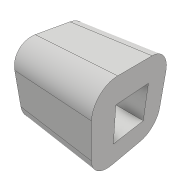
# Autodesk Inventor part: Winding
Saved by Autodesk Inventor 2018.2 (Build 222227000, 227)
## iProperties
Created: 2019-02-04
Part Number: Winding
Material: Generic
Document SubType Name: Modeling
Designer: ns6022
Density: 1 g/cm^3
Appearance: Default
Author: ns6022
Autodesk Inventor part; units mm, degrees
ref_plane "YZ Plane" through (0, 0, 0) normal (1, 0, 0) x (0, 1, 0)
ref_plane "XZ Plane" through (0, 0, 0) normal (0, 1, 0) x (-1, 0, 0)
ref_plane "XY Plane" through (0, 0, 0) normal (0, 0, 1) x (1, 0, 0)
sketch "Sketch1" plane through (0, 0, 0) normal (0, 0, 1) x (1, 0, 0)
  point P0 (0, 0)
sketch "LAYER1" plane through (0, 0, 0) normal (0, 0, 1) x (1, 0, 0)
  line L0 (70, 20.5) -> (90, 20.5)
  line L1 (90, 20.5) -> (90, 57.5)
  line L2 (90, 57.5) -> (0, 57.5)
  line L3 (0, 57.5) -> (0, -57.5)
  line L4 (0, -57.5) -> (90, -57.5)
  line L5 (90, -57.5) -> (90, -20.5)
  line L6 (90, -20.5) -> (70, -20.5)
  line L7 (70, -20.5) -> (70, -37.5)
  line L8 (70, -37.5) -> (20, -37.5)
  line L9 (20, -37.5) -> (20, 37.5)
  line L10 (20, 37.5) -> (70, 37.5)
  line L11 (70, 37.5) -> (70, 20.5)
  constraints: 24 end point
sketch "LAYER2" plane through (0, 0, 0) normal (0, 0, 1) x (1, 0, 0)
  line L0 (20.1, -20) -> (110.1, -20)
  line L1 (110.1, -20) -> (110.1, 20)
  line L2 (110.1, 20) -> (20.1, 20)
  line L3 (20.1, 20) -> (20.1, -20)
  constraints: 8 end point
sketch "LAYER3" plane through (0, 0, 0) normal (0, 0, 1) x (1, 0, 0)
  line L0 (20.5, -71.2) -> (69.5, -71.2)
  line L1 (69.5, -71.2) -> (69.5, -58)
  line L2 (69.5, -58) -> (20.5, -58)
  line L3 (20.5, -58) -> (20.5, -71.2)
  constraints: 8 end point
sketch "LAYER4" plane through (0, 0, 0) normal (0, 0, 1) x (1, 0, 0)
  line L0 (20.5, -23.8) -> (69.5, -23.8)
  line L1 (69.5, -23.8) -> (69.5, -37)
  line L2 (69.5, -37) -> (20.5, -37)
  line L3 (20.5, -37) -> (20.5, -23.8)
  constraints: 8 end point
sketch "LAYER5" plane through (0, 0, 0) normal (0, 0, 1) x (1, 0, 0)
  line L0 (20.5, 23.8) -> (69.5, 23.8)
  line L1 (69.5, 23.8) -> (69.5, 37)
  line L2 (69.5, 37) -> (20.5, 37)
  line L3 (20.5, 37) -> (20.5, 23.8)
  constraints: 8 end point
sketch "LAYER6" plane through (0, 0, 0) normal (0, 0, 1) x (1, 0, 0)
  line L0 (20.5, 71.2) -> (69.5, 71.2)
  line L1 (69.5, 71.2) -> (69.5, 58)
  line L2 (69.5, 58) -> (20.5, 58)
  line L3 (20.5, 58) -> (20.5, 71.2)
  constraints: 8 end point
extrude "Extrusion3" add sketch "LAYER3" along normal blind 47.4
extrude "Extrusion4" add sketch "LAYER4" along normal blind 47.4
sketch "Sketch9" plane through (20.5, -37, 0) normal (-1, 0, 0) x (0, 0, 1)
  line L0 (0, 0) -> (47.4, 0) projected
  line L1 (0, -21) -> (47.4, -21) projected
  line L2 (47.4, 0) -> (47.4, -21)
  line L3 (0, 0) -> (0, -21)
  line L4 (13.2, 0) -> (13.2, -21)
  line L5 (34.2, 0) -> (34.2, -21)
  point P0 (0, 37)
  dimension "d12" = 13.2
  dimension "d13" = 13.2
  constraints: 8 end point, 4 point on line, 3 parallel, 1 perpendicular
  measures "d12" distance between parallel lines of L5 L2
  measures "d13" distance between parallel lines of L3 L4
extrude "Extrusion6" add sketch "Sketch9" against normal up to surface (49 mm away) contours L0 L4 L1 L3 | L0 L2 L1 L5
fillet "Fillet1" radius 13.2 4 edges at (45, -23.8, 47.4) (45, -71.2, 47.4) (45, -71.2, 0) (45, -23.8, 0)
body "Solid3"
